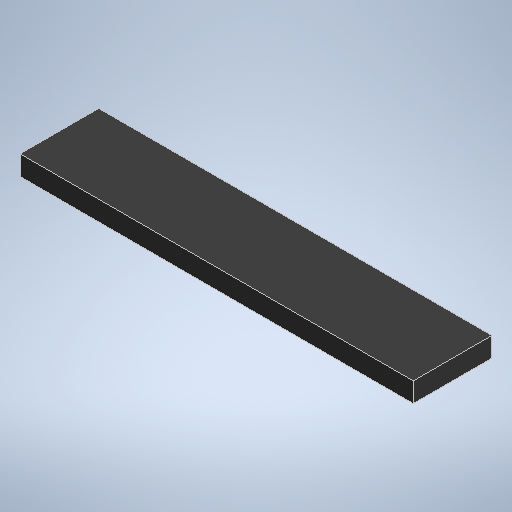
# Autodesk Inventor part: Stopper
Saved by Autodesk Inventor 2025 (Build 290162010, 162A)
## iProperties
Created: 2024-11-26
Part Number: Stopper
Material: Gummi, Silikon(1)
Document SubType Name: Modeling
Designer: Admin
Density: 1.25 g/cm^3
Appearance: Gummi - Schwarz(2)
Author: Admin
Autodesk Inventor part; units mm, degrees
ref_plane "YZ Plane" through (0, 0, 0) normal (1, 0, 0) x (0, 1, 0)
ref_plane "XZ Plane" through (0, 0, 0) normal (0, 1, 0) x (-1, 0, 0)
ref_plane "XY Plane" through (0, 0, 0) normal (0, 0, 1) x (1, 0, 0)
sketch "Skizze1" plane through (0, 0, 0) normal (0, 0, 1) x (1, 0, 0)
  line L0 (58.2721, 12.4722) -> (38.2721, 12.4722)
  line L1 (38.2721, 12.4722) -> (38.2721, 16.4722)
  line L2 (38.2721, 16.4722) -> (58.2721, 16.4722)
  line L3 (58.2721, 16.4722) -> (58.2721, 12.4722)
  point P0 (0, 0)
  dimension "d0" = 20
  dimension "d1" = 4
  constraints: 8 end point, 2 parallel, 1 horizontal, 1 perpendicular
  measures "d0" distance of L1.end L2.end
  measures "d1" distance of L0.end L1.end
extrude "Extrusion1" add sketch "Skizze1" along normal blind 1
